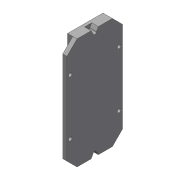
# Autodesk Inventor part: BC-10008_B
Saved by Autodesk Inventor 2016 (Build 200138000, 138)
## iProperties
Created: 2015-09-23
Part Number: BC-10008_B
Project: Xxxxxxxxxx xxxxxxxxx XXX
Cost Center: 0.00.00.000
Material: Aço Carbono
Document SubType Name: Modeling
Designer: Reinaldo.Basílio
Density: 7.87 g/cm^3
Appearance: Steel
Mass: 9311.68 g
Surface Area: 1319.11 cm^2
Volume: 1183.19 cm^3
RuleStatus: InUse
AfterMaterialChange0: file://_iMaterial
AfterAnyiPropertyChange0: file://_iMaterial
AfterDocNew0: file://_Naming_par
AfterDocNew1: file://_NameStart
AfterDocNew2: file://_NameStart1
AfterDocNew3: file://_Materiais
DocNumber: XXXXX-XXX-XXXX-00-001.ipt
Folder: .
Title: SSD
Author: Reinaldo.Basílio
Autodesk Inventor part; units mm, degrees
ref_plane "YZ Plane" through (0, 0, 0) normal (1, 0, 0) x (0, 1, 0)
ref_plane "XZ Plane" through (0, 0, 0) normal (0, 1, 0) x (-1, 0, 0)
ref_plane "XY Plane" through (0, 0, 0) normal (0, 0, 1) x (1, 0, 0)
sketch "Sketch5" plane through (0, 0, 0) normal (0, 1, 0) x (-1, 0, 0)
  line L0 (52.5, -165) -> (52.5, 165)
  line L1 (-52.5, 165) -> (52.5, 165)
  line L2 (-52.5, -165) -> (-52.5, 165)
  line L3 (52.5, -165) -> (-52.5, -165)
  point P0 (0, 0)
  point P1 (0, 0)
  point P2 (70, 0)
  dimension "d8" = 330
  dimension "d9" = 105
  dimension "d26" = 52.5
  dimension "d27" = 165
  constraints: 8 end point, 2 horizontal, 2 vertical
  measures "d8" distance of L2.start L1.start
  measures "d9" distance of L1.start L0.end
  measures "d26" distance from line of L0 point (0, 0)
  measures "d27" distance from line of L1 point (0, 0)
extrude "Extrusion5" add sketch "Sketch5" along normal blind 15.5
sketch "Sketch6" plane through (0, 15.5, 0) normal (0, 1, 0) x (1, 0, 0)
  line L0 (-52.5, -165) -> (52.5, -165)
  circle A0 centre (0, -155) radius 5
  line L1 (52.5, 165) -> (-52.5, 165)
  circle A1 centre (0, 155) radius 5
  line L2 (-52.5, 165) -> (-52.5, -165) projected
  line L3 (-52.5, -165) -> (52.5, -165) projected
  line L4 (52.5, -165) -> (52.5, 165) projected
  line L5 (52.5, 165) -> (-52.5, 165) projected
  point P0 (0, -165)
  dimension "d12" = 10
  dimension "d20" = 10
  dimension "d21" = 10
  constraints: 4 end point, 2 centre point, 2 vertical alignment, 1 equal radius, 1 midpoint
  measures "d12" distance from line of L0 A0.centre
  measures "d20" distance from line of L1 A1.centre
  measures "d21" diameter of A0
hole "Hole1" at (0, 15.5, 155) at (0, 15.5, -155) direction (0, -1, 0) diameter 10 depth 7
sketch "Sketch7" plane through (0, 15.5, 0) normal (0, 1, 0) x (1, 0, 0)
  circle A0 centre (0, -155) radius 5
  line L0 (-52.5, 165) -> (-52.5, -165)
  line L1 (-52.5, -165) -> (52.5, -165)
  line L2 (5, -155) -> (-5, -155)
  line L3 (5, -155) -> (10.7735, -165)
  line L4 (-5, -155) -> (-10.7735, -165)
  line L5 (0, -155) -> (0, -162.7031)
  line L6 (10.7735, -165) -> (-10.7735, -165)
  line L7 (-52.5, 0) -> (15.6822, 0)
  line L8 (5, 155) -> (-5, 155)
  line L9 (5, 155) -> (10.7735, 165)
  line L10 (-5, 155) -> (-10.7735, 165)
  line L11 (0, 155) -> (0, 162.7031)
  line L12 (10.7735, 165) -> (-10.7735, 165)
  circle A1 centre (0, -155) radius 5 projected
  circle A2 centre (0, 155) radius 5 projected
  line L13 (-52.5, 165) -> (-52.5, -165) projected
  line L14 (-52.5, -165) -> (52.5, -165) projected
  line L15 (52.5, -165) -> (52.5, 165) projected
  line L16 (52.5, 165) -> (-52.5, 165) projected
  dimension "d22" = 60
  dimension "d23" = 30
  constraints: 26 end point, 7 symmetric about line, 5 midpoint, 2 horizontal, 2 point on circle, 2 point on line, 1 centre point, 1 coincident, 1 collinear, 1 vertical
  measures "d22" angle of L3 L4
  measures "d23" angle of L3 L5
extrude "Extrusion6" cut sketch "Sketch7" against normal blind 7 contours L3 L1 L4 A0 | A0 L5 L2 | L2 L5 A0 | L9 A2 L10 L12 | L8 L11 A2 | L8 A2 L11
sketch "Sketch8" plane through (0, 15.5, 0) normal (0, 1, 0) x (1, 0, 0)
  line L0 (10.7735, 165) -> (5, 155) projected
  arc A0 (-5, 155) -> (5, 155) centre (0, 155) ccw projected
  line L1 (-5, 155) -> (-10.7735, 165) projected
  line L2 (-10.7735, 165) -> (-52.5, 165) projected
  line L3 (-52.5, 165) -> (-52.5, -165) projected
  line L4 (-52.5, -165) -> (-10.7735, -165) projected
  line L5 (-10.7735, -165) -> (-5, -155) projected
  arc A1 (5, -155) -> (-5, -155) centre (0, -155) ccw projected
  line L6 (5, -155) -> (10.7735, -165) projected
  line L7 (10.7735, -165) -> (52.5, -165) projected
  line L8 (52.5, -165) -> (52.5, 165) projected
  line L9 (52.5, 165) -> (10.7735, 165) projected
  line L10 (82.5, 165) -> (82.5, -165)
  line L11 (-82.5, -165) -> (-82.5, 165)
  line L12 (52.5, -165) -> (82.5, -165)
  line L13 (-52.5, -165) -> (-82.5, -165)
  line L14 (-52.5, 165) -> (-82.5, 165)
  line L15 (52.5, 165) -> (82.5, 165)
  point P0 (0, 0)
  dimension "d28" = 30
  dimension "d29" = 30
  constraints: 12 end point, 2 horizontal, 1 perpendicular
  measures "d28" distance between parallel lines of L11 L3
  measures "d29" distance between parallel lines of L10 L8
extrude "Extrusion7" add sketch "Sketch8" along normal blind 12.5
chamfer "Chamfer1" distance 30 angle 45 4 edges at (82.5, 21.75, 165) (-82.5, 21.75, 165) (82.5, 21.75, -165) (-82.5, 21.75, -165)
sketch "Sketch10" plane through (0, 28, 0) normal (0, 1, 0) x (1, 0, 0)
  arc A0 (5, -155) -> (-5, -155) centre (0, -155) ccw projected
  circle A1 centre (-72.5, -82.5) radius 5.25
  circle A2 centre (-72.5, 82.5) radius 5.25
  line L0 (0, 0) -> (0, -14.0329) construction
  circle A3 centre (72.5, -82.5) radius 5.25
  circle A4 centre (72.5, 82.5) radius 5.25
  dimension "d36" = 10.5
  dimension "d37" = 72.5
  dimension "d38" = 165
  dimension "d39" = 82.5
  constraints: 4 centre point, 2 end point, 2 symmetric about line, 1 equal radius, 1 vertical, 1 vertical alignment, 2 other
  measures "d36" diameter of A1
  measures "d37" horizontal distance of A1.centre A0.centre
  measures "d38" distance of A2.centre A1.centre
  measures "d39" vertical distance of L0.start A1.centre
hole "Hole2" at (-72.5, 28, 82.5) at (72.5, 28, 82.5) at (72.5, 28, -82.5) at (-72.5, 28, -82.5) direction (0, -1, 0) diameter 10.5 end through all
sketch "Sketch11" plane through (0, 28, 0) normal (0, 1, 0) x (1, 0, 0)
  circle A0 centre (0, 155) radius 1.7421
  arc A1 (-5, 155) -> (5, 155) centre (0, 155) ccw projected
  circle A2 centre (76.6339, -81.1985) radius 4
  line L0 (0, 155) -> (0, -122.4158)
  circle A3 centre (72.5, 82.5) radius 5.25 projected
  circle A4 centre (-72.5, -82.5) radius 5.25 projected
  circle A5 centre (-72.5, 82.5) radius 5.25 projected
  line L1 (-82.5, 135) -> (-52.5, 165) projected
  line L2 (-82.5, 135) -> (-82.5, -135) projected
  line L3 (-52.5, -165) -> (-82.5, -135) projected
  line L4 (-52.5, -165) -> (-10.7735, -165) projected
  line L5 (-10.7735, -165) -> (-5, -155) projected
  arc A6 (5, -155) -> (-5, -155) centre (0, -155) ccw projected
  line L6 (5, -155) -> (10.7735, -165) projected
  line L7 (10.7735, -165) -> (52.5, -165) projected
  line L8 (82.5, -135) -> (52.5, -165) projected
  line L9 (82.5, -135) -> (82.5, 135) projected
  line L10 (52.5, 165) -> (82.5, 135) projected
  line L11 (52.5, 165) -> (10.7735, 165) projected
  line L12 (10.7735, 165) -> (5, 155) projected
  line L13 (-5, 155) -> (-10.7735, 165) projected
  line L14 (-10.7735, 165) -> (-52.5, 165) projected
  line L15 (64.5, 127.5442) -> (64.5, -127.5442)
  line L16 (0, 155) -> (72.5, -82.5)
  line L17 (76.6483, -77.1986) -> (67.3477, -77.1986)
  line L18 (80.6339, -81.2093) -> (80.6339, -74.4951)
  circle A7 centre (72.5, -82.5) radius 4
  circle A8 centre (68.344, -83.7291) radius 4
  line L19 (78.8574, -87.7291) -> (66.6744, -87.7291)
  circle A9 centre (72.5, -82.5) radius 5.25 projected
  line L20 (-82.5, 0) -> (-62.0923, 0)
  dimension "d59" = 8
  dimension "d65" = 18
  dimension "d66" = 12
  dimension "d68" = 248.3193
  dimension "d71" = 8
  dimension "d72" = 8
  dimension "d73" = 4.156
  dimension "d74" = 10.5306
  dimension "d75" = 8.1339
  dimension "d76" = 82.5
  constraints: 14 end point, 4 centre point, 3 horizontal, 2 point on circle, 2 vertical, 1 coincident, 1 concentric, 1 midpoint, 1 tangent
  measures "d59" diameter of A2
  measures "d65" distance between parallel lines of L9 L15
  measures "d66" distance from line of L7.end L15
  measures "d68" distance of A2.centre A0.centre
  measures "d71" diameter of A7
  measures "d72" diameter of A8
  measures "d73" horizontal distance of A8.centre A7.centre
  measures "d74" distance between parallel lines of L17 L19
  measures "d75" distance from line of L18 L16.end
  measures "d76" distance from line of A7.centre L20
sketch "Sketch13" plane through (0, 15.5, 0) normal (0, -1, 0) x (1, 0, 0)
  circle A0 centre (-72.5, 82.5) radius 5.25 projected
  circle A1 centre (-72.5, -82.5) radius 5.25 projected
  circle A2 centre (-72.5, 82.5) radius 7.5
  circle A3 centre (-72.5, -82.5) radius 7.5
  line L0 (0, 0) -> (0, -18.6046)
  circle A4 centre (72.5, 82.5) radius 7.5
  circle A5 centre (72.5, -82.5) radius 7.5
  circle A6 centre (72.5, 82.5) radius 5.25
  circle A7 centre (72.5, -82.5) radius 5.25
  dimension "d77" = 15
  constraints: 6 centre point, 4 symmetric about line, 2 coincident, 2 end point, 1 equal radius, 1 vertical, 4 other
  measures "d77" diameter of A2
hole "Hole3" at (-72.5, 15.5, 82.5) at (72.5, 15.5, 82.5) at (72.5, 15.5, -82.5) at (-72.5, 15.5, -82.5) direction (0, 1, 0) diameter 15 depth 0.5
equation "\"d26\" = 0.5 * d9"
equation "\"d27\" = 0.5 * d8"
equation "\"d20\" = d12"
equation "\"d23\" = 0.5 * d22"
equation "\"d29\" = d28"
equation "\"d39\" = 0.5 * d38"
body "Solid5"
